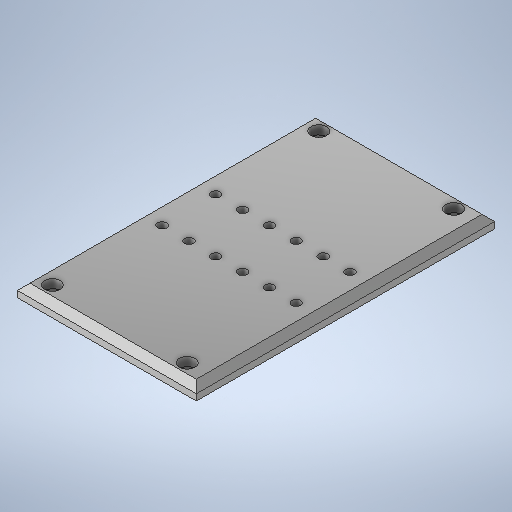
# Autodesk Inventor part: Mounting Plate
Saved by Autodesk Inventor 2025 (Build 290162000, 162)
## iProperties
Created: 2024-08-16
Part Number: Mounting Plate
Material: Aluminum 6061
Document SubType Name: Modeling
Designer: Caleb Fangmeier
Density: 2.7 g/cm^3
Appearance: Anodized - Light Gray
Author: Caleb Fangmeier
Autodesk Inventor part; units mm, degrees
ref_plane "YZ Plane" through (0, 0, 0) normal (1, 0, 0) x (0, 1, 0)
ref_plane "XZ Plane" through (0, 0, 0) normal (0, 1, 0) x (-1, 0, 0)
ref_plane "XY Plane" through (0, 0, 0) normal (0, 0, 1) x (1, 0, 0)
sketch "Sketch1" plane through (0, 0, 0) normal (0, 1, 0) x (-1, 0, 0)
  line L0 (-45, -75) -> (45, -75)
  line L1 (45, -75) -> (45, 75)
  line L2 (45, 75) -> (-45, 75)
  line L3 (-45, 75) -> (-45, -75)
  line L4 (-45, -75) -> (45, 75) construction
  line L5 (45, -75) -> (-45, 75) construction
  point P0 (0, 0)
  dimension "d0" = 150
  dimension "d1" = 90
  constraints: 12 end point, 2 midpoint, 2 parallel, 1 horizontal, 1 perpendicular
  measures "d0" distance of L0.end L1.end
  measures "d1" distance of L1.end L2.end
extrude "Extrusion1" add sketch "Sketch1" along normal blind 6.35
chamfer "Chamfer1" distance 3.175 angle 45 4 edges at (45, 6.35, 0) (0, 6.35, 75) (-45, 6.35, 0) (0, 6.35, -75)
sketch "Sketch3" plane through (0, 6.35, 0) normal (0, 1, 0) x (1, 0, 0)
  line L0 (-45, -75) -> (45, -75) projected
  line L1 (-45, 75) -> (-45, -75) projected
  line L2 (45, -75) -> (45, 75) projected
  line L3 (45, 75) -> (-45, 75) projected
  point P0 (0, 0)
  point P1 (-35.4, -67)
  point P2 (-35.4, 67)
  point P3 (32.4, 67)
  point P4 (32.4, -67)
  dimension "d7" = 9.6
  dimension "d8" = 8
  dimension "d9" = 8
  dimension "d10" = 12.6
  constraints: 2 horizontal alignment, 2 vertical alignment
  measures "d7" distance from line of L1 point (-35.4, -67)
  measures "d8" distance from line of L0 point (-35.4, -67)
  measures "d9" distance from line of L3 point (-35.4, 67)
  measures "d10" distance from line of L2 point (32.4, -67)
hole "Hole1" at (-35.4, 6.35, 67) at (-35.4, 6.35, -67) at (32.4, 6.35, -67) at (32.4, 6.35, 67) direction (0, -1, 0) diameter 4.7 depth 7.9 tip angle 118 counterbore diameter 7.9 counterbore depth 4.4
sketch "Sketch4" plane through (0, 0, 0) normal (0, -1, 0) x (1, 0, 0)
  line L0 (45, -75) -> (-45, -75) projected
  point P0 (0, 0)
  point P1 (-33.75, -13.5)
  point P2 (-33.75, 13.5)
  point P3 (-20.25, 13.5)
  point P4 (-20.25, -13.5)
  point P5 (-6.75, 13.5)
  point P6 (-6.75, -13.5)
  point P7 (6.75, 13.5)
  point P8 (6.75, -13.5)
  point P9 (20.25, 13.5)
  point P10 (20.25, -13.5)
  point P11 (33.75, 13.5)
  point P12 (33.75, -13.5)
  dimension "d18" = 27
  dimension "d19" = 13.5
  dimension "d22" = 13.5
  dimension "d34" = 6.75
  constraints: 1 horizontal, 1 vertical alignment, 10 other
  measures "d18" distance of point (-33.75, -13.5) point (-33.75, 13.5)
  measures "d19" vertical distance of point (0, 0) point (-33.75, 13.5)
  measures "d22" distance of point (-33.75, 13.5) point (-20.25, 13.5)
  measures "d34" horizontal distance of point (0, 0) point (6.75, -13.5)
hole "Hole2" at (-33.75, 0, -13.5) at (-33.75, 0, 13.5) at (-20.25, 0, 13.5) at (-20.25, 0, -13.5) at (-6.75, 0, 13.5) at (-6.75, 0, -13.5) at (6.75, 0, 13.5) at (6.75, 0, -13.5) at (20.25, 0, 13.5) at (20.25, 0, -13.5) at (33.75, 0, 13.5) at (33.75, 0, -13.5) direction (0, 1, 0) diameter 4.5 depth 7.9 tip angle 118 countersink diameter 9.4 countersink angle 90 clearance for "Flat Head Machine Screw" size "M4" standard "Ansi Metric M Profile"
equation "\"d9\" = d8"
equation "\"d19\" = 0.5 * d18"
equation "\"d34\" = 0.5 * d19"
body "Solid1"
